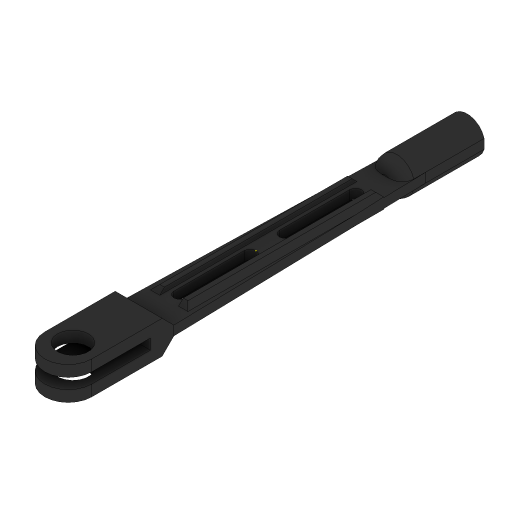
# Autodesk Inventor part: link2_long_print
Saved by Autodesk Inventor 2023 (Build 270158000, 158)
## iProperties
Created: 2023-11-03
Part Number: link2_long_print
Material: Ogólny
Document SubType Name: Modeling
Designer: janek
Density: 1 g/cm^3
Appearance: Domyślna
Author: janek
## iProperties of the stored document link2_print_Drukowanie 3D.ipt
Created: 2023-11-13
Part Number: link2_print_Drukowanie 3D
Material: Ogólny
Document SubType Name: Modeling
Designer: janek
Density: 1 g/cm^3
Appearance: Domyślna
Author: janek
Autodesk Inventor part; units mm, degrees
ref_plane "YZ Plane" through (0, 0, 0) normal (1, 0, 0) x (0, 1, 0)
ref_plane "XZ Plane" through (0, 0, 0) normal (0, 1, 0) x (-1, 0, 0)
ref_plane "XY Plane" through (0, 0, 0) normal (0, 0, 1) x (1, 0, 0)
sketch "Szkic1" plane through (0, 0, 0) normal (0, 1, 0) x (-1, 0, 0)
  line L0 (10, 90) -> (-10, 90)
  line L1 (-10, 90) -> (-10, -90)
  line L2 (-10, -90) -> (10, -90)
  line L3 (10, -90) -> (10, 90)
  line L4 (10, 90) -> (-10, -90) construction
  line L5 (-10, 90) -> (10, -90) construction
  point P0 (0, 0)
  dimension "d0" = 20
  dimension "d1" = 180
  constraints: 12 end point, 2 midpoint, 2 parallel, 1 horizontal, 1 perpendicular
  measures "d0" distance of L2.end L1.end
  measures "d1" distance between parallel lines of L2 L0
extrude "Wyciągnięcie proste1" add sketch "Szkic1" along normal blind 4
sketch "Szkic2" plane through (0, 4, 0) normal (0, 1, 0) x (1, 0, 0)
  circle A0 centre (0, -80) radius 2
  line L0 (-10, -90) -> (10, -90) projected
  point P0 (0, 0)
  dimension "d4" = 4
  dimension "d5" = 10
  constraints: 1 centre point
  measures "d4" diameter of A0
  measures "d5" distance from line of L0 A0.centre
extrude "Wyciągnięcie proste2" cut sketch "Szkic2" against normal blind 4
sketch "Szkic4" plane through (0, 4, 0) normal (0, 1, 0) x (1, 0, 0)
  line L0 (-10, -90) -> (10, -90) projected
  line L1 (-10, 90) -> (-10, -90) projected
  line L2 (10, -90) -> (-10, -90)
  line L3 (-10, -90) -> (-10, -45)
  line L4 (-10, -45) -> (10, -45)
  line L5 (10, -45) -> (10, -90)
  point P0 (0, 0)
  dimension "d9" = 45
  constraints: 8 end point, 2 parallel, 1 horizontal, 1 perpendicular, 1 point on line
  measures "d9" distance from line of L4 L0.end
extrude "Wyciągnięcie proste3" add sketch "Szkic4" along normal blind 5
sketch "Szkic5" plane through (0, 0, 0) normal (0, -1, 0) x (1, 0, 0)
  line L0 (-10, 90) -> (10, 90) projected
  line L1 (10, 90) -> (10, -90) projected
  line L2 (-10, 90) -> (10, 90)
  line L3 (10, 90) -> (10, 45)
  line L4 (10, 45) -> (-10, 45)
  line L5 (-10, 45) -> (-10, 90)
  point P0 (0, 0)
  point P1 (0, 45)
  point P2 (0, 90)
  dimension "d12" = 45
  constraints: 8 end point, 2 midpoint, 2 parallel, 1 horizontal, 1 perpendicular, 1 point on line
  measures "d12" distance of point (0, 45) point (0, 90)
extrude "Wyciągnięcie proste4" add sketch "Szkic5" along normal blind 5
sketch "Szkic6" plane through (-10, 0, -90) normal (-1, 0, 0) x (0, 0, 1)
  line L0 (180, 9) -> (180, -5) projected
  line L1 (180, -0.25) -> (145, -0.25)
  line L2 (145, -0.25) -> (145, 4.25)
  line L3 (145, 4.25) -> (180, 4.25)
  line L4 (180, 4.25) -> (180, -0.25)
  line L5 (135, 9) -> (180, 9) projected
  point P0 (90, 0)
  point P1 (180, 4.25)
  dimension "d15" = 35
  dimension "d16" = 4.5
  dimension "d17" = 4.75
  constraints: 8 end point, 2 parallel, 1 horizontal, 1 perpendicular, 1 point on line
  measures "d15" distance of L2.end L3.end
  measures "d16" distance between parallel lines of L3 L1
  measures "d17" distance between parallel lines of L5 L3
extrude "Wyciągnięcie proste5" cut sketch "Szkic6" against normal blind 29
sketch "Szkic7" plane through (0, -5, 0) normal (0, -1, 0) x (1, 0, 0)
  circle A0 centre (0, 78) radius 6.6
  line L0 (10, 90) -> (-10, 90) projected
  point P0 (0, 0)
  point P1 (0, 90)
  dimension "d20" = 13.2
  dimension "d23" = 12
  constraints: 1 centre point, 1 midpoint
  measures "d20" diameter of A0
  measures "d23" distance of point (0, 90) A0.centre
extrude "Wyciągnięcie proste6" cut sketch "Szkic7" against normal blind 29
sketch "Szkic8" plane through (10, 0, -90) normal (0, 0, -1) x (-1, 0, 0)
  circle A0 centre (10, 2) radius 7.5
  line L0 (0, 4) -> (20, 4) projected
  line L1 (0, 0) -> (0, 4) projected
  point P0 (10, 0)
  point P1 (10, 4)
  dimension "d24" = 15
  dimension "d25" = 2
  dimension "d26" = 10
  constraints: 1 centre point, 1 midpoint
  measures "d24" diameter of A0
  measures "d25" distance of A0.centre point (10, 4)
  measures "d26" distance from line of L1 A0.centre
extrude "Wyciągnięcie proste7" add sketch "Szkic8" against normal blind 25
fillet "Zaokrąglenie1" radius 10 4 edges at (10, 6.625, 90) (10, -2.625, 90) (-10, 6.625, 90) (-10, -2.625, 90)
chamfer "Faza1" distance 5 angle 45 1 edges at (0, -5, 45)
chamfer "Faza2" distance 5 angle 45 1 edges at (0, 9, 45)
sketch "Szkic10" plane through (-10, 0, -90) normal (0, 0, -1) x (-1, 0, 0)
  circle A0 centre (-10, 2) radius 4.75
  line L0 (0, 0) -> (0, 4) projected
  line L1 (0, 9) -> (-20, 9) projected
  point P0 (-10, 0)
  point P1 (0, 2)
  dimension "d42" = 9.5
  dimension "d43" = 10
  dimension "d44" = 7
  constraints: 1 centre point, 1 midpoint
  measures "d42" diameter of A0
  measures "d43" distance of point (0, 2) A0.centre
  measures "d44" distance from line of L1 A0.centre
extrude "Wyciągnięcie proste9" cut sketch "Szkic10" against normal blind 17
sketch "Szkic11" plane through (0, 0, 0) normal (0, -1, 0) x (1, 0, 0)
  line L0 (-7.2284, -90) -> (7.2284, -90) projected
  line L1 (10, 45) -> (10, -90) projected
  line L2 (7.2284, -90) -> (10, -90)
  line L3 (10, -90) -> (10, -65)
  line L4 (10, -65) -> (7.2284, -65)
  line L5 (7.2284, -65) -> (7.2284, -90)
  line L6 (-10, -90) -> (-10, 45) projected
  line L7 (-7.2284, -65) -> (-7.2284, -90) projected
  line L8 (-10, -90) -> (-7.2284, -90)
  line L9 (-7.2284, -90) -> (-7.2284, -65)
  line L10 (-7.2284, -65) -> (-10, -65)
  line L11 (-10, -65) -> (-10, -90)
  point P0 (0, 0)
  point P1 (8.6142, -90)
  point P2 (8.6142, -65)
  point P3 (-10, -65)
  dimension "d47" = 25
  constraints: 16 end point, 4 parallel, 2 horizontal, 2 midpoint, 2 perpendicular, 1 point on line
  measures "d47" distance of point (8.614, -90) point (8.614, -65)
extrude "Wyciągnięcie proste10" cut sketch "Szkic11" against normal blind 20
sketch "Szkic12" plane through (0, 4, 0) normal (0, 1, 0) x (1, 0, 0)
  point P0 (0, 0)
sketch "Szkic13" plane through (10, 0, -65) normal (0, 0, 1) x (1, 0, 0)
  line L0 (0, 4) -> (-2.7716, 4) projected
  line L1 (-2.7716, 4) -> (-17.2284, 4) projected
  arc A0 (-2.7716, 4) -> (-17.2284, 4) centre (-10, 2) ccw
  point P0 (-10, 0)
  constraints: 2 point on circle, 1 centre point
extrude "Wyciągnięcie proste11" add sketch "Szkic13" along normal blind 10
fillet "Zaokrąglenie2" radius 5 1 edges at (0, 9.5, -55)
sketch "Szkic14" plane through (10, 0, -65) normal (0, 0, 1) x (1, 0, 0)
  line L0 (-17.2284, 0) -> (-2.7716, 0) projected
  arc A0 (-17.2284, 0) -> (-2.7716, 0) centre (-10, 2) ccw
  circle A1 centre (-10, 2) radius 4.75 projected
  point P0 (-10, 0)
  constraints: 2 point on circle, 1 centre point, 1 concentric
extrude "Wyciągnięcie proste12" add sketch "Szkic14" along normal blind 10 contours L0 A1 A0 | L0 A1 picked at (-11.249, -0.3064)
fillet "Zaokrąglenie3" radius 5 1 edges at (0, -5.5, -55)
chamfer "Faza3" distance 110 distance2 2.75 1 edges at (-10, 2, -65) measured on face at (-10, 1.3333, -28.3333)
chamfer "Faza4" distance 110 distance2 2.75 1 edges at (10, 2, -65) measured on face at (10, 2.6667, -28.3333)
sketch "Szkic15" plane through (0, 0, 0) normal (0, -1, 0) x (1, 0, 0)
  line L0 (4, -45) -> (6, -45)
  line L1 (6, -45) -> (6, 35)
  line L2 (6, 35) -> (4, 35)
  line L3 (4, 35) -> (4, -45)
  line L4 (-6, -45) -> (-4, -45)
  line L5 (-4, -45) -> (-4, 35)
  line L6 (-4, 35) -> (-6, 35)
  line L7 (-6, 35) -> (-6, -45)
  arc A0 (2.5, 32.5) -> (-2.5, 32.5) centre (0, 32.5) ccw projected
  arc A1 (-2.5, -42.5) -> (2.5, -42.5) centre (0, -42.5) ccw projected
  line L8 (2.5, 32.5) -> (2.5, -42.5) projected
  line L9 (-2.5, -42.5) -> (-2.5, 32.5) projected
  line L10 (0, -45) -> (0, -10) construction
  line L11 (-2.5, -42.5) -> (-2.5, -12.5)
  line L12 (2.5, -12.5) -> (2.5, -42.5)
  arc A2 (-2.5, -42.5) -> (2.5, -42.5) centre (0, -42.5) ccw
  arc A3 (2.5, -12.5) -> (-2.5, -12.5) centre (0, -12.5) ccw
  line L13 (0, 35) -> (0, 0) construction
  line L14 (-2.5, 32.5) -> (-2.5, 2.5)
  line L15 (2.5, 2.5) -> (2.5, 32.5)
  arc A4 (2.5, 32.5) -> (-2.5, 32.5) centre (0, 32.5) ccw
  arc A5 (-2.5, 2.5) -> (2.5, 2.5) centre (0, 2.5) ccw
  point P0 (0, 0)
  point P1 (5, 35)
  point P2 (5, -45)
  point P3 (0, -27.5)
  point P4 (0, 17.5)
  point P5 (0, -10)
  point P6 (0, -45)
  point P7 (0, 35)
  point P8 (0, 0)
  dimension "d62" = 0
  dimension "d63" = 0
  dimension "d64" = 1.5
  dimension "d65" = 1.5
  dimension "d66" = 2
  dimension "d67" = 2
  dimension "d68" = 35
  dimension "d69" = 35
  constraints: 32 end point, 18 point on circle, 8 parallel, 8 tangent, 6 point on line, 4 centre point, 4 midpoint, 2 horizontal, 2 perpendicular
  measures "d62" vertical distance of L13.start point (5, 35)
  measures "d63" vertical distance of L10.start point (5, -45)
  measures "d64" distance between parallel lines of L8 L3
  measures "d65" distance between parallel lines of L5 L9
  measures "d66" distance between parallel lines of L5 L7
  measures "d67" distance between parallel lines of L3 L1
  measures "d68" distance of point (0, -10) point (0, -45)
  measures "d69" distance of point (0, 35) point (0, 0)
extrude "Wyciągnięcie proste14" cut sketch "Szkic15" against normal blind 5 contours L8 A5 L9 A0 | L8 A1 L9 A3
extrude "Wyciągnięcie proste15" add sketch "Szkic15" along normal blind 2 contours L3 L2 L1 L0 | L7 L6 L5 L4
sketch "Szkic16" plane through (0, 4, 0) normal (0, 1, 0) x (1, 0, 0)
  line L0 (6, -35) -> (6, 45) projected
  line L1 (4, 45) -> (4, -35) projected
  line L2 (6, 45) -> (4, 45)
  line L3 (4, 45) -> (4, -35)
  line L4 (4, -35) -> (6, -35)
  line L5 (6, -35) -> (6, 45)
  line L6 (-4, -35) -> (-4, 45) projected
  line L7 (-6, -35) -> (-6, 45) projected
  line L8 (-4, 45) -> (-6, 45)
  line L9 (-6, 45) -> (-6, -35)
  line L10 (-6, -35) -> (-4, -35)
  line L11 (-4, -35) -> (-4, 45)
  point P0 (0, 0)
  constraints: 16 end point, 4 parallel, 2 horizontal, 2 perpendicular
extrude "Wyciągnięcie proste16" add sketch "Szkic16" along normal blind 2
chamfer "Faza5" distance 2 angle 45 12 edges at (-6, 0, -5) (6, 0, -5) (-6, 4, -5) (6, 4, -5) (5, 4, 35) (-5, 4, 35) (5, 4, -45) (-5, 4, -45) (-5, 0, -45) (5, 0, -45) (-5, 0, 35) (5, 0, 35)
